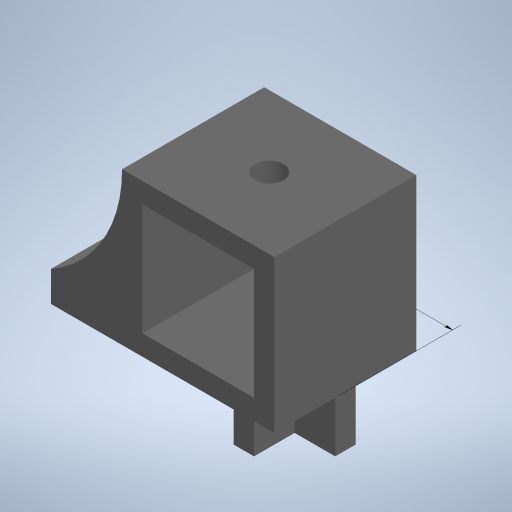
# Autodesk Inventor part: position_setter_normal
Saved by Autodesk Inventor 2024.1 (Build 281209000, 209)
## iProperties
Created: 2025-09-28
Part Number: position_setter_normal
Material: 一般
Document SubType Name: Modeling
Designer: hibik
Density: 1 g/cm^3
Appearance: 既定
Author: hibik
Autodesk Inventor part; units mm, degrees
ref_plane "YZ Plane" through (0, 0, 0) normal (1, 0, 0) x (0, 1, 0)
ref_plane "XZ Plane" through (0, 0, 0) normal (0, 1, 0) x (-1, 0, 0)
ref_plane "XY Plane" through (0, 0, 0) normal (0, 0, 1) x (1, 0, 0)
sketch "スケッチ1" plane through (0, 0, 0) normal (0, 0, 1) x (1, 0, 0)
  line L0 (5.5, -5.5) -> (-5.5, -5.5)
  line L1 (-5.5, -5.5) -> (-5.5, 5.5)
  line L2 (-5.5, 5.5) -> (5.5, 5.5)
  line L3 (5.5, 5.5) -> (5.5, -5.5)
  line L4 (5.5, -5.5) -> (-5.5, 5.5) construction
  line L5 (-5.5, -5.5) -> (5.5, 5.5) construction
  line L6 (7.5, -7.5) -> (-7.5, -7.5)
  line L7 (-7.5, -7.5) -> (-7.5, 7.5)
  line L8 (-7.5, 7.5) -> (7.5, 7.5)
  line L9 (7.5, 7.5) -> (7.5, -7.5)
  line L10 (7.5, -7.5) -> (-7.5, 7.5) construction
  line L11 (-7.5, -7.5) -> (7.5, 7.5) construction
  point P0 (0, 0)
  dimension "d0" = 11
  dimension "d1" = 11
  dimension "d2" = 2
  constraints: 24 end point, 4 midpoint, 4 parallel, 2 horizontal, 2 perpendicular, 1 collinear
  measures "d0" distance of L1.end L2.end
  measures "d1" distance of L0.end L1.end
  measures "d2" distance between parallel lines of L9 L3
extrude "押し出し1" add sketch "スケッチ1" along normal blind 14
sketch "スケッチ2" plane through (0, 0, 14) normal (0, 0, 1) x (1, 0, 0)
  line L0 (-7.5, 7.5) -> (-7.5, -7.5) projected
  line L1 (-7.5, -7.5) -> (-14.5, -7.5)
  line L2 (-14.5, -7.5) -> (-14.5, -4.5)
  line L3 (-14.5, -4.5) -> (-7.5, -4.5)
  line L4 (-7.5, -4.5) -> (-7.5, -7.5)
  arc A0 (-14.5, -4.5) -> (-7.5, 7.5) centre (-21.2857, 7.5) ccw
  point P0 (0, 0)
  dimension "d5" = 7
  dimension "d6" = 3
  constraints: 8 end point, 2 parallel, 2 point on circle, 1 centre point, 1 horizontal, 1 perpendicular, 1 tangent
  measures "d5" distance of L2.end L3.end
  measures "d6" distance of L1.end L2.end
extrude "押し出し2" add sketch "スケッチ2" against normal up to surface (14 mm away)
sketch "スケッチ3" plane through (7.5, 7.5, 14) normal (0, 1, 0) x (1, 0, 0)
  circle A0 centre (-7.5, 7) radius 1.4
  line L0 (0, 14) -> (0, 0) projected
  line L1 (0, 14) -> (-15, 14) projected
  point P0 (-7.5, 14)
  point P1 (0, 7)
  point P2 (-7.5, 14)
  dimension "d9" = 2.8
  constraints: 2 midpoint, 1 centre point, 1 horizontal alignment, 1 vertical alignment
  measures "d9" diameter of A0
extrude "押し出し3" cut sketch "スケッチ3" against normal up to surface (2 mm away)
sketch "スケッチ4" plane through (7.5, -7.5, 0) normal (0, -1, 0) x (1, 0, 0)
  line L0 (-6, 12) -> (-4, 12)
  line L1 (-4, 12) -> (-4, 2)
  line L2 (-4, 2) -> (-6, 2)
  line L3 (-6, 2) -> (-6, 12)
  line L4 (-10, 8) -> (0, 8)
  line L5 (0, 8) -> (0, 6)
  line L6 (0, 6) -> (-10, 6)
  line L7 (-10, 6) -> (-10, 8)
  line L8 (0, 0) -> (0, 14) projected
  point P0 (-7.5, 0)
  point P1 (0, 7)
  point P2 (0, 7)
  point P3 (-5, 12)
  point P4 (-5, 8)
  point P5 (-6, 7)
  point P6 (-10, 7)
  point P7 (-6, 8)
  point P8 (-6, 6)
  point P9 (-4, 6)
  point P10 (-4, 8)
  dimension "d12" = 10
  dimension "d13" = 2
  constraints: 16 end point, 6 midpoint, 4 parallel, 4 perpendicular, 2 horizontal, 1 coincident, 1 collinear, 1 horizontal alignment, 1 vertical alignment
  measures "d12" distance of L4.start L4.end
  measures "d13" distance of L0.start L0.end
extrude "押し出し4" add sketch "スケッチ4" along normal blind 5
sketch "スケッチ5" plane through (7.5, 7.5, 14) normal (0, 1, 0) x (1, 0, 0)
  line L0 (-15.3, 8.3568) -> (-15.3, 5.6432)
  line L1 (-15.3, 5.6432) -> (-17.65, 4.2865)
  line L2 (-17.65, 4.2865) -> (-20, 5.6432)
  line L3 (-20, 5.6432) -> (-20, 8.3568)
  line L4 (-20, 8.3568) -> (-17.65, 9.7135)
  line L5 (-17.65, 9.7135) -> (-15.3, 8.3568)
  circle A0 centre (-17.65, 7) radius 1.6
  line L6 (-22, 0) -> (-22, 14) projected
  point P0 (-7.5, 14)
  point P1 (-20, 7)
  point P2 (-22, 7)
  dimension "d16" = 4.7
  dimension "d17" = 3.2
  dimension "d24" = 2
  constraints: 12 end point, 2 midpoint, 1 centre point, 1 coincident, 1 horizontal alignment, 13 other
  measures "d16" distance from line of point (-20, 7) L0
  measures "d17" diameter of A0
  measures "d24" distance between parallel lines of L6 L3
extrude "押し出し5" cut sketch "スケッチ5" against normal through all contours A0
extrude "押し出し6" cut sketch "スケッチ5" against normal up to surface (13 mm away) contours L0 L1 L2 L3 L4 L5 | A0
